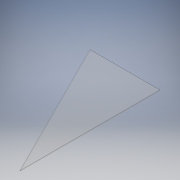
# Autodesk Inventor part: Plexi-SideV!
Saved by Autodesk Inventor 2019 (Build 230136000, 136)
## iProperties
Created: 2021-09-16
Part Number: Plexi-SideV!
Material: Acrylic, Clear
Document SubType Name: Modeling
Designer: timmy
Density: 1.19 g/cm^3
Appearance: Transparent - Clear
Author: timmy
Autodesk Inventor part; units mm, degrees
ref_plane "YZ Plane" through (0, 0, 0) normal (1, 0, 0) x (0, 1, 0)
ref_plane "XZ Plane" through (0, 0, 0) normal (0, 1, 0) x (-1, 0, 0)
ref_plane "XY Plane" through (0, 0, 0) normal (0, 0, 1) x (1, 0, 0)
sketch "Sketch5" plane through (0, 0, 0) normal (1, 0, 0) x (0, 1, 0)
  line L0 (0, 0) -> (152.4, 0) construction
  line L1 (152.4, 0) -> (152.4, -914.4)
  line L2 (152.4, -914.4) -> (0, -914.4) construction
  line L3 (0, -914.4) -> (0, 0) construction
  line L4 (152.4, 0) -> (609.6, -457.2)
  line L5 (152.4, 0) -> (798.9784, 0) construction
  line L6 (609.6, -457.2) -> (152.4, -914.4)
  dimension "d18" = 45
  constraints: 14 end point, 2 horizontal, 2 parallel, 1 equal length, 1 perpendicular
  measures "d18" angle of L4 L5
extrude "Extrusion5" add sketch "Sketch5" along normal blind 3.175
body "Solid3"
